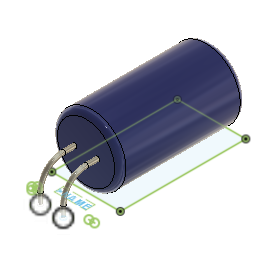
Capacitor-6X11-E-FLAT v4 (Autodesk Fusion 360 design; units mm, degrees)
Autodesk Fusion 360 part; units mm, degrees
ref_plane "WorkPlane1" through (0, 3, 0) normal (0, 1, 0) x (0, 0, 1)
sketch "Sketch1" plane through (0, 3, 0) normal (0, 1, 0) x (1, 0, 0)
  circle A0 centre (0, -3) radius 3
  dimension "d2" = 6
  dimension "d3" = 3
  measures "d2" diameter of A0
  measures "d3" distance of origin A0.centre
extrude "Extrude1" add sketch "Sketch1" along normal blind 11
ref_plane "WorkPlane2" through (1, 0, 0) normal (1, 0, 0) x (0, 1, 0)
sketch "Sketch2" plane through (1, 0, 0) normal (1, 0, 0) x (0, 1, 0)
  line L0 (0, 0) -> (0, 1)
  line L1 (2, 3) -> (3, 3)
  arc A0 (2, 3) -> (0, 1) centre (2, 1) ccw
  line L2 (3, 0) -> (14, 0)
  dimension "d7" = 2
  dimension "d8" = 3
  constraint coincident L0.start origin
  constraint vertical L0
  constraint perpendicular L0 L1
  constraint tangent L0 A0
  constraint tangent L1 A0
  measures "d7" radius of A0
  measures "d8" distance of L1 L2
sketch "Sketch3" plane through (0, 0, 0) normal (0, 0, 1) x (1, 0, 0)
  circle A0 centre (1, 0) radius 0.2
  dimension "d9" = 0.4
  measures "d9" diameter of A0
pipe "Pipe1" add diameter 0.4 path "Sketch2" along L0 A0 L1
mirror "Mirror1" about plane through (0, 0, 0) normal (1, 0, 0) of "Pipe1"
fillet "Fillet1" radius 0.5 1 faces at (2.9963, 10.3333, 3.1495)
